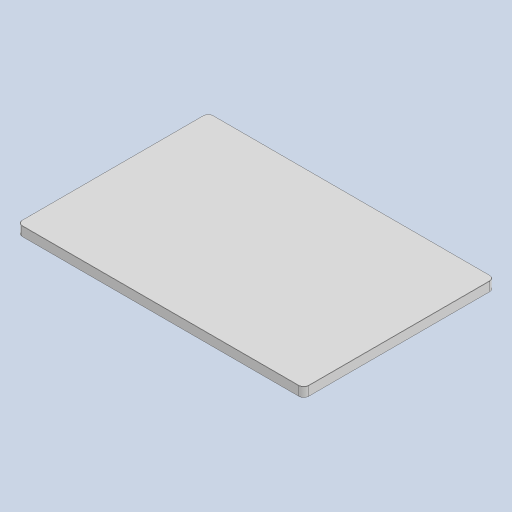
# Autodesk Inventor part: readDataFromDB
Saved by Autodesk Inventor 2023 (Build 270158000, 158)
## iProperties
Created: 2023-07-25
Part Number: readDataFromDB
Material: Generic
Document SubType Name: Modeling
Designer: pkrol
Density: 1 g/cm^3
Appearance: Default
Author: pkrol
Autodesk Inventor part; units mm, degrees
ref_plane "YZ Plane" through (0, 0, 0) normal (1, 0, 0) x (0, 1, 0)
ref_plane "XZ Plane" through (0, 0, 0) normal (0, 1, 0) x (-1, 0, 0)
ref_plane "XY Plane" through (0, 0, 0) normal (0, 0, 1) x (1, 0, 0)
sketch "Sketch1" plane through (0, 0, 0) normal (0, 1, 0) x (-1, 0, 0)
  line L0 (-600, -400) -> (600, -400)
  line L1 (600, -400) -> (600, 400)
  line L2 (600, 400) -> (-600, 400)
  line L3 (-600, 400) -> (-600, -400)
  line L4 (-600, -400) -> (600, 400) construction
  line L5 (600, -400) -> (-600, 400) construction
  point P0 (0, 0)
  dimension "height" = 1200
  dimension "width" = 800
  constraints: 12 end point, 2 midpoint, 2 parallel, 1 horizontal, 1 perpendicular
  measures "height" distance of L1.end L2.end
  measures "width" distance of L0.end L1.end
extrude "Extrusion1" add sketch "Sketch1" along normal blind 40
fillet "Fillet1" radius 20 4 edges at (600, 20, -400) (600, 20, 400) (-600, 20, 400) (-600, 20, -400)
chamfer "Chamfer3" distance 1 angle 45 16 edges at (600, 0, 0) (594.1421, 0, -394.1421) (0, 0, -400) (-594.1421, 0, -394.1421) (-600, 0, 0) (-594.1421, 0, 394.1421) (0, 0, 400) (594.1421, 0, 394.1421) (600, 40, 0) (594.1421, 40, -394.1421) (0, 40, -400) (-594.1421, 40, -394.1421) (-600, 40, 0) (-594.1421, 40, 394.1421) (0, 40, 400) (594.1421, 40, 394.1421)
equation "\"height\" = height_user"
equation "\"width\" = width_user"
equation "\"thickness\" = thickness_user"
equation "\"radius\" = radius_user"
equation "\"chamfer\" = chamfer_user"
equation "\"height_user\" = 1200"
equation "\"width_user\" = 800"
equation "\"thickness_user\" = 40"
equation "\"chamfer_user\" = 1"
equation "\"radius_user\" = 20"
body "Solid1"
